Autodesk Inventor part; units mm, degrees
(part 3 of 3)
extrude "Vysunutí10" cut sketch "Náčrt5" against normal up to next contours L13 L12 L11 L10 | L33 L32 L31 L30 | L37 L39 L38 L36 | L43 L45 L44 L42 | L49 L51 L50 L48 | L55 L57 L56 L54 | L61 L63 L62 L60 | L67 L69 L68 L66 | L73 L75 L74 L72 | L79 L81 L80 L78 | L85 L87 L86 L84 | L91 L93 L92 L90 | L97 L99 L98 L96 | L103 L105 L104 L102 | L109 L111 L110 L108 | L115 L117 L116 L114 | L121 L123 L122 L120 | L127 L129 L128 L126 | L133 L135 L134 L132 | L139 L141 L140 L138 | L145 L147 L146 L144 | L151 L153 L152 L150 | L157 L159 L158 L156 | L163 L165 L164 L162 | L169 L171 L170 L168 | L175 L177 L176 L174 | L181 L183 L182 L180 | L187 L189 L188 L186 | L193 L195 L194 L192 | L199 L201 L200 L198 | L205 L207 L206 L204 | L211 L213 L212 L210 | L217 L219 L218 L216 | L223 L225 L224 L222 | L229 L231 L230 L228 | L235 L237 L236 L234 | L241 L243 L242 L240 | L247 L249 L248 L246 | L253 L255 L254 L252 | L259 L261 L260 L258 | L265 L267 L266 L264 | L271 L273 L272 L270 | L277 L279 L278 L276 | L283 L285 L284 L282 | L289 L291 L290 L288 | L295 L297 L296 L294 | L301 L303 L302 L300 | L307 L309 L308 L306 | L313 L315 L314 L312 | L319 L321 L320 L318 | L325 L327 L326 L324 | L331 L333 L332 L330 | L337 L339 L338 L336 | L343 L345 L344 L342 | L349 L351 L350 L348 | L355 L357 L356 L354 | L361 L363 L362 L360 | L367 L369 L368 L366 | L373 L375 L374 L372 | L379 L381 L380 L378 | L385 L387 L386 L384 | L391 L393 L392 L390 | L397 L399 L398 L396 | L403 L405 L404 L402 | L409 L411 L410 L408 | L417 L416 L415 L414 | L422 L423 L421 L420 | L428 L429 L427 L426 | L434 L435 L433 L432 | L440 L441 L439 L438 | L446 L447 L445 L444 | L452 L453 L451 L450 | L458 L459 L457 L456 | L464 L465 L463 L462 | L470 L471 L469 L468 | L476 L477 L475 L474 | L482 L483 L481 L480 | L488 L489 L487 L486 | L494 L495 L493 L492 | L500 L501 L499 L498 | L506 L507 L505 L504 | L512 L513 L511 L510 | L518 L519 L517 L516 | L524 L525 L523 L522 | L530 L531 L529 L528 | L536 L537 L535 L534 | L542 L543 L541 L540 | L548 L549 L547 L546 | L554 L555 L553 L552 | L560 L561 L559 L558 | L566 L567 L565 L564 | L572 L573 L571 L570 | L578 L579 L577 L576 | L584 L585 L583 L582 | L590 L591 L589 L588 | L596 L597 L595 L594 | L602 L603 L601 L600 | L608 L609 L607 L606 | L614 L615 L613 L612 | L620 L621 L619 L618 | L626 L627 L625 L624 | L632 L633 L631 L630 | L638 L639 L637 L636 | L644 L645 L643 L642 | L650 L651 L649 L648 | L656 L657 L655 L654 | L662 L663 L661 L660 | L668 L669 L667 L666 | L674 L675 L673 L672 | L680 L681 L679 L678 | L686 L687 L685 L684 | L692 L693 L691 L690 | L698 L699 L697 L696 | L704 L705 L703 L702 | L710 L711 L709 L708 | L716 L717 L715 L714 | L722 L723 L721 L720 | L728 L729 L727 L726 | L734 L735 L733 L732 | L740 L741 L739 L738 | L746 L747 L745 L744 | L752 L753 L751 L750 | L758 L759 L757 L756 | L764 L765 L763 L762 | L770 L771 L769 L768 | L776 L777 L775 L774 | L782 L783 L781 L780 | L788 L789 L787 L786 | L794 L795 L793 L792 | L800 L799 L803 L798 | L806 L805 L809 L804 | L812 L811 L815 L810 | L818 L817 L821 L816 | L824 L823 L827 L822 | L830 L829 L833 L828 | L836 L835 L839 L834 | L842 L841 L845 L840 | L848 L847 L851 L846 | L854 L853 L857 L852 | L860 L859 L863 L858 | L866 L865 L869 L864 | L872 L871 L875 L870 | L878 L877 L881 L876 | L884 L883 L887 L882 | L890 L889 L893 L888 | L896 L895 L899 L894 | L902 L901 L905 L900 | L908 L907 L911 L906 | L914 L913 L917 L912 | L920 L919 L923 L918 | L926 L925 L929 L924 | L932 L931 L935 L930 | L938 L937 L941 L936 | L944 L943 L947 L942 | L950 L949 L953 L948 | L956 L955 L959 L954 | L962 L961 L965 L960 | L968 L967 L971 L966 | L974 L973 L977 L972 | L980 L979 L983 L978 | L986 L985 L989 L984 | L992 L991 L995 L990 | L998 L997 L1001 L996 | L1004 L1003 L1007 L1002 | L1010 L1009 L1013 L1008 | L1016 L1015 L1019 L1014 | L1022 L1021 L1025 L1020 | L1028 L1027 L1031 L1026 | L1034 L1033 L1037 L1032 | L1040 L1039 L1043 L1038 | L1046 L1045 L1049 L1044 | L1052 L1051 L1055 L1050 | L1058 L1057 L1061 L1056 | L1064 L1063 L1067 L1062 | L1070 L1069 L1073 L1068 | L1076 L1075 L1079 L1074 | L1082 L1081 L1085 L1080 | L1088 L1087 L1091 L1086 | L1094 L1093 L1097 L1092 | L1100 L1099 L1103 L1098 | L1106 L1105 L1109 L1104 | L1112 L1111 L1115 L1110 | L1118 L1117 L1121 L1116 | L1124 L1123 L1127 L1122 | L1130 L1129 L1133 L1128 | L1136 L1135 L1139 L1134 | L1142 L1141 L1145 L1140 | L1148 L1147 L1151 L1146 | L1154 L1153 L1157 L1152 | L1160 L1159 L1163 L1158 | L1166 L1165 L1169 L1164 | L1172 L1171 L1175 L1170 | L1180 L1181 L1182 L1183 | L1184 L1185 L1186 L1187 | L1188 L1189 L1190 L1191 | L1192 L1193 L1194 L1195 | L1196 L1197 L1198 L1199 | L1200 L1201 L1202 L1203 | L1204 L1205 L1206 L1207 | L1208 L1209 L1210 L1211 | L1212 L1213 L1214 L1215 | L1216 L1217 L1218 L1219 | L1220 L1221 L1222 L1223 | L1224 L1225 L1226 L1227 | L1228 L1229 L1230 L1231 | L1232 L1233 L1234 L1235 | L1236 L1237 L1238 L1239 | L1240 L1241 L1242 L1243 | L1244 L1245 L1246 L1247 | L1248 L1249 L1250 L1251 | L1252 L1253 L1254 L1255 | L1256 L1257 L1258 L1259 | L1260 L1261 L1262 L1263 | L1264 L1265 L1266 L1267 | L1268 L1269 L1270 L1271 | L1272 L1273 L1274 L1275 | L1276 L1277 L1278 L1279 | L1280 L1281 L1282 L1283 | L1284 L1285 L1286 L1287 | L1288 L1289 L1290 L1291 | L1292 L1293 L1294 L1295 | L1296 L1297 L1298 L1299 | L1300 L1301 L1302 L1303 | L1304 L1305 L1306 L1307 | L1308 L1309 L1310 L1311 | L1312 L1313 L1314 L1315 | L1316 L1317 L1318 L1319 | L1320 L1321 L1322 L1323 | L1324 L1325 L1326 L1327 | L1328 L1329 L1330 L1331 | L1332 L1333 L1334 L1335 | L1336 L1337 L1338 L1339 | L1340 L1341 L1342 L1343 | L1344 L1345 L1346 L1347 | L1348 L1349 L1350 L1351 | L1352 L1353 L1354 L1355 | L1356 L1357 L1358 L1359 | L1360 L1361 L1362 L1363 | L1364 L1365 L1366 L1367 | L1368 L1369 L1370 L1371 | L1372 L1373 L1374 L1375 | L1376 L1377 L1378 L1379 | L1380 L1381 L1382 L1383 | L1384 L1385 L1386 L1387 | L1388 L1389 L1390 L1391 | L1392 L1393 L1394 L1395 | L1396 L1397 L1398 L1399 | L1400 L1401 L1402 L1403 | L1404 L1405 L1406 L1407 | L1408 L1409 L1410 L1411 | L1412 L1413 L1414 L1415 | L1416 L1417 L1418 L1419 | L1420 L1421 L1422 L1423 | L1424 L1425 L1426 L1427 | L1428 L1429 L1430 L1431 | L1432 L1433 L1434 L1435
sketch "Náčrt10" plane through (0, 2.54, 0) normal (0, 1, 0) x (1, 0, 0)
  line L0 (40.64, -167.64) -> (-40.64, -167.64)
  line L1 (-40.64, -167.64) -> (-40.64, -172.72)
  line L2 (-40.64, -172.72) -> (40.64, -172.72)
  line L3 (40.64, -172.72) -> (40.64, -167.64)
  line L4 (40.64, -167.64) -> (-40.64, -172.72) construction
  line L5 (-40.64, -167.64) -> (40.64, -172.72) construction
  line L6 (-248.92, 0) -> (248.92, 0) projected
  line L7 (0, 248.92) -> (0, -248.92) projected
  line L8 (-177.8, -177.8) -> (177.8, -177.8) projected
  line L9 (40.64, 167.64) -> (-40.64, 167.64)
  line L10 (-40.64, 167.64) -> (-40.64, 172.72)
  line L11 (-40.64, 172.72) -> (40.64, 172.72)
  line L12 (40.64, 172.72) -> (40.64, 167.64)
  line L13 (40.64, 167.64) -> (-40.64, 172.72) construction
  line L14 (-40.64, 167.64) -> (40.64, 172.72) construction
  line L15 (-167.64, 40.64) -> (-172.72, 40.64)
  line L16 (-172.72, 40.64) -> (-172.72, -40.64)
  line L17 (-172.72, -40.64) -> (-167.64, -40.64)
  line L18 (-167.64, -40.64) -> (-167.64, 40.64)
  line L19 (-167.64, 40.64) -> (-172.72, -40.64) construction
  line L20 (-172.72, 40.64) -> (-167.64, -40.64) construction
  line L21 (-177.8, 177.8) -> (-177.8, -177.8) projected
  line L22 (167.64, 40.64) -> (172.72, 40.64)
  line L23 (172.72, 40.64) -> (172.72, -40.64)
  line L24 (172.72, -40.64) -> (167.64, -40.64)
  line L25 (167.64, -40.64) -> (167.64, 40.64)
  line L26 (167.64, 40.64) -> (172.72, -40.64) construction
  line L27 (172.72, 40.64) -> (167.64, -40.64) construction
  line L28 (66.04, -166.37) -> (66.04, -167.005)
  line L29 (66.04, -167.005) -> (66.675, -167.005)
  line L30 (66.675, -167.005) -> (66.675, -166.37)
  line L31 (66.675, -166.37) -> (66.04, -166.37)
  line L32 (66.04, -166.37) -> (66.675, -167.005) construction
  line L33 (66.04, -167.005) -> (66.675, -166.37) construction
  line L34 (69.215, -166.37) -> (68.58, -166.37)
  line L35 (68.58, -166.37) -> (68.58, -167.005)
  line L36 (69.215, -167.005) -> (69.215, -166.37)
  line L37 (68.58, -166.37) -> (69.215, -167.005) construction
  line L38 (68.58, -167.005) -> (69.215, -167.005)
  line L39 (68.58, -167.005) -> (69.215, -166.37) construction
  line L40 (71.755, -166.37) -> (71.12, -166.37)
  line L41 (71.12, -166.37) -> (71.12, -167.005)
  line L42 (71.755, -167.005) -> (71.755, -166.37)
  line L43 (71.12, -166.37) -> (71.755, -167.005) construction
  line L44 (71.12, -167.005) -> (71.755, -167.005)
  line L45 (71.12, -167.005) -> (71.755, -166.37) construction
  line L46 (74.295, -166.37) -> (73.66, -166.37)
  line L47 (73.66, -166.37) -> (73.66, -167.005)
  line L48 (74.295, -167.005) -> (74.295, -166.37)
  line L49 (73.66, -166.37) -> (74.295, -167.005) construction
  line L50 (73.66, -167.005) -> (74.295, -167.005)
  line L51 (73.66, -167.005) -> (74.295, -166.37) construction
  line L52 (76.835, -166.37) -> (76.2, -166.37)
  line L53 (76.2, -166.37) -> (76.2, -167.005)
  line L54 (76.835, -167.005) -> (76.835, -166.37)
  line L55 (76.2, -166.37) -> (76.835, -167.005) construction
  line L56 (76.2, -167.005) -> (76.835, -167.005)
  line L57 (76.2, -167.005) -> (76.835, -166.37) construction
  line L58 (66.675, -163.83) -> (66.04, -163.83)
  line L59 (66.04, -163.83) -> (66.04, -164.465)
  line L60 (66.675, -164.465) -> (66.675, -163.83)
  line L61 (66.04, -163.83) -> (66.675, -164.465) construction
  line L62 (66.04, -164.465) -> (66.675, -164.465)
  line L63 (66.04, -164.465) -> (66.675, -163.83) construction
  line L64 (69.215, -163.83) -> (68.58, -163.83)
  line L65 (68.58, -163.83) -> (68.58, -164.465)
  line L66 (69.215, -164.465) -> (69.215, -163.83)
  line L67 (68.58, -163.83) -> (69.215, -164.465) construction
  line L68 (68.58, -164.465) -> (69.215, -164.465)
  line L69 (68.58, -164.465) -> (69.215, -163.83) construction
  line L70 (71.755, -163.83) -> (71.12, -163.83)
  line L71 (71.12, -163.83) -> (71.12, -164.465)
  line L72 (71.755, -164.465) -> (71.755, -163.83)
  line L73 (71.12, -163.83) -> (71.755, -164.465) construction
  line L74 (71.12, -164.465) -> (71.755, -164.465)
  line L75 (71.12, -164.465) -> (71.755, -163.83) construction
  line L76 (74.295, -163.83) -> (73.66, -163.83)
  line L77 (73.66, -163.83) -> (73.66, -164.465)
  line L78 (74.295, -164.465) -> (74.295, -163.83)
  line L79 (73.66, -163.83) -> (74.295, -164.465) construction
  line L80 (73.66, -164.465) -> (74.295, -164.465)
  line L81 (73.66, -164.465) -> (74.295, -163.83) construction
  line L82 (76.835, -163.83) -> (76.2, -163.83)
  line L83 (76.2, -163.83) -> (76.2, -164.465)
  line L84 (76.835, -164.465) -> (76.835, -163.83)
  line L85 (76.2, -163.83) -> (76.835, -164.465) construction
  line L86 (76.2, -164.465) -> (76.835, -164.465)
  line L87 (76.2, -164.465) -> (76.835, -163.83) construction
  point P0 (0, 0)
  point P1 (0, -170.18)
  point P2 (0, 170.18)
  point P3 (-170.18, 0)
  point P4 (170.18, 0)
  point P5 (66.3575, -166.6875)
  point P6 (68.8975, -166.6875)
  point P7 (71.4375, -166.6875)
  point P8 (73.9775, -166.6875)
  point P9 (76.5175, -166.6875)
  point P10 (66.3575, -164.1475)
  point P11 (68.8975, -164.1475)
  point P12 (71.4375, -164.1475)
  point P13 (73.9775, -164.1475)
  point P14 (76.5175, -164.1475)
  dimension "d191" = 2.54
  dimension "d194" = 2.54
  dimension "d172" = 81.28
  dimension "d173" = 5.08
  dimension "d174" = 0
  dimension "d175" = 5.08
  dimension "d176" = 0
  dimension "d177" = 5.08
  dimension "d188" = 0.635
  dimension "d198" = 10.795
  dimension "d199" = 25.4
  dimension "d202" = 2.54
  dimension "d205" = 2.54
  constraints: 168 end point, 28 midpoint, 10 symmetric about line, 6 parallel, 6 perpendicular, 4 horizontal, 2 vertical, 99 other
  measures "d172" distance of L1.end L2.end
  measures "d173" distance of L2.end L0.start
  measures "d174" distance from line of L7 point (0, -170.18)
  measures "d175" distance between parallel lines of L8 L2
  measures "d176" distance from line of L6 point (-170.18, 0)
  measures "d177" distance between parallel lines of L21 L16
  measures "d188" distance of L29.end L30.end
  measures "d198" distance between parallel lines of L8 L29
  measures "d199" distance between parallel lines of L3 L28
  measures "d202" distance of L30.end L34.start
  measures "d205" distance of L30.end L58.start
extrude "Vysunutí11" [suppressed]
equation "\"d2\" = pcbOuterSize"
equation "\"d3\" = pcbOuterSize"
equation "\"d4\" = pcbInnerSize"
equation "\"d5\" = pcbInnerSize"
equation "\"d6\" = pinHeaderPinDist"
equation "\"d18\" = 0.5 * wireDist"
equation "\"d19\" = wireDia"
equation "\"d20\" = wireLen"
equation "\"d12\" = wireDia"
equation "\"d35\" = wireDia"
equation "\"d36\" = wireLen"
equation "\"d37\" = 0.5 * wireDist"
equation "\"d39\" = wireDia"
equation "\"d23\" = wireDist"
equation "\"d43\" = wireDist"
equation "\"pcbOuterSize\" = 355.6"
equation "\"pcbInnerSize\" = 254"
equation "\"pinHeaderPinDist\" = 2.54"
equation "\"wireDist\" = 7.62"
equation "\"wireDia\" = 0.2"
equation "\"wireLen\" = 17.78"
